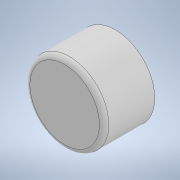
# Autodesk Inventor part: buttonForCatButton
Saved by Autodesk Inventor 2021.2 (Build 252289000, 289)
## iProperties
Created: 2020-11-25
Part Number: buttonForCatButton
Material: Generic
Document SubType Name: Modeling
Designer: robst
Density: 1 g/cm^3
Appearance: Default
Author: robst
Autodesk Inventor part; units mm, degrees
ref_plane "YZ Plane" through (0, 0, 0) normal (1, 0, 0) x (0, 1, 0)
ref_plane "XZ Plane" through (0, 0, 0) normal (0, 1, 0) x (-1, 0, 0)
ref_plane "XY Plane" through (0, 0, 0) normal (0, 0, 1) x (1, 0, 0)
sketch "Sketch1" plane through (0, 0, 0) normal (0, 0, 1) x (1, 0, 0)
  circle A0 centre (0, 0) radius 8.89
  dimension "d0" = 17.78
  constraints: 1 centre point, 1 coincident
  measures "d0" diameter of A0
extrude "Extrusion1" add sketch "Sketch1" against normal blind 11.43
sketch "Sketch2" plane through (0, 0, -11.43) normal (0, 0, -1) x (-1, 0, 0)
  circle A0 centre (0, 0) radius 5.5245
  dimension "d3" = 11.049
  constraints: 1 centre point, 1 coincident
  measures "d3" diameter of A0
extrude "Extrusion2" cut sketch "Sketch2" against normal blind 3.81
fillet "Fillet1" radius 1.0583 1 edges at (-8.89, 0, 0)
ref_plane "Work Plane1" through (0, 0, -8.89) normal (0, 0, -1) x (-1, 0, 0)
sketch "Sketch3" plane through (0, 0, -8.89) normal (0, 0, -1) x (-1, 0, 0)
  circle A0 centre (0, 0) radius 0.635
  dimension "d8" = 1.27
  constraints: 1 centre point, 1 coincident
  measures "d8" diameter of A0
loft "Loft1" add profiles "Sketch3" section 1 edges at (5.5245, 0, -7.62)
sketch "Sketch4" plane through (0, 0, -8.89) normal (0, 0, -1) x (-1, 0, 0)
  circle A0 centre (0, 0) radius 0.635 projected
  circle A1 centre (0, 0) radius 0.9525
  dimension "d13" = 1.905
  constraints: 1 centre point, 1 coincident
  measures "d13" diameter of A1
extrude "Extrusion3" cut sketch "Sketch4" against normal blind 1.27 contours A0
equation "\"d0\" = outsideDiameterForHoleInCat"
equation "\"d1\" = length"
equation "\"d3\" = holeForInteriorButton"
equation "\"d4\" = depthForInteriorButton"
equation "\"d6\" = topFilletRadius"
equation "\"d8\" = offsetCircleDiameter"
equation "\"d13\" = glueHoleDiameter"
equation "\"d14\" = glueHoleDepth"
equation "\"outsideDiameterForHoleInCat\" = 17.78"
equation "\"length\" = 11.43"
equation "\"holeForInteriorButton\" = 11.049"
equation "\"depthForInteriorButton\" = 3.81"
equation "\"planeOffset\" = 0.635"
equation "\"offsetCircleDiameter\" = 1.27"
equation "\"topFilletRadius\" = 1.05833"
equation "\"glueHoleDiameter\" = 1.905"
equation "\"glueHoleDepth\" = 1.27"
body "Solid1"
